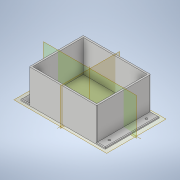
# Autodesk Inventor part: Box
Saved by Autodesk Inventor 2021 (Build 250183000, 183)
## iProperties
Created: 2024-05-07
Part Number: Box
Material: Generisch
Document SubType Name: Modeling
Designer: pasca
Density: 1 g/cm^3
Appearance: Vorgabe
Author: pasca
Autodesk Inventor part; units mm, degrees
sketch "Skizze1" plane through (0, 0, 0) normal (0, 0, 1) x (1, 0, 0)
  line L0 (-100, 80) -> (100, 80)
  line L1 (100, 80) -> (100, -80)
  line L2 (100, -80) -> (-100, -80)
  line L3 (-100, -80) -> (-100, 80)
  line L4 (0, -112) -> (0, 112) projected
  line L5 (-140, 0) -> (140, 0) projected
  point P0 (0, 0)
  dimension "d0" = 160
  dimension "d1" = 200
  constraints: 8 end point, 2 parallel, 1 horizontal, 1 perpendicular, 2 other
  measures "d0" distance between parallel lines of L2 L0
  measures "d1" distance between parallel lines of L1 L3
extrude "Extrusion1" add sketch "Skizze1" along normal blind 100
sketch "Skizze2" plane through (0, 0, 100) normal (0, 0, 1) x (1, 0, 0)
  line L0 (-95, 75) -> (95, 75)
  line L1 (95, 75) -> (95, -75)
  line L2 (95, -75) -> (-95, -75)
  line L3 (-95, -75) -> (-95, 75)
  line L4 (0, -112) -> (0, 112) projected
  line L5 (-140, 0) -> (140, 0) projected
  point P0 (0, 0)
  dimension "d4" = 150
  dimension "d5" = 190
  constraints: 8 end point, 2 parallel, 1 horizontal, 1 perpendicular, 2 other
  measures "d4" distance between parallel lines of L2 L0
  measures "d5" distance between parallel lines of L1 L3
extrude "Extrusion2" cut sketch "Skizze2" against normal blind 95
sketch "Skizze3" plane through (0, 0, 5) normal (0, 0, 1) x (1, 0, 0)
  line L0 (100, -80) -> (100, 80) projected
  line L1 (100, -80) -> (125, -80)
  line L2 (125, -80) -> (125, 80)
  line L3 (125, 80) -> (100, 80)
  line L4 (100, 80) -> (100, -80)
  point P0 (0, 0)
  constraints: 8 end point, 2 parallel, 1 horizontal, 1 perpendicular
extrude "Extrusion3" add sketch "Skizze3" against normal blind 5
sketch "Skizze4" plane through (0, 0, 5) normal (0, 0, 1) x (1, 0, 0)
  point P0 (0, 0)
sketch "Skizze5" plane through (0, 0, 5) normal (0, 0, 1) x (1, 0, 0)
  line L0 (100, -80) -> (100, 80) projected
  line L1 (100, -80) -> (125, -80) projected
  line L2 (125, -80) -> (125, 80) projected
  line L3 (125, 80) -> (100, 80) projected
  point P0 (0, 0)
  point P1 (112.5, 55)
  point P2 (112.5, -55)
hole "Bohrung2" at (112.5, 55, 5) at (112.5, -55, 5) direction (0, 0, -1) diameter 6.4 depth 8 tip angle 118
mirror "Spiegeln1" about plane through (0, 0, 0) normal (1, 0, 0) of "Extrusion3", "Bohrung2"
fillet "Rundung1" radius 2 10 edges at (125, 0, 5) (-125, 0, 5) (-112.5, -80, 5) (-100, -80, 52.5) (112.5, -80, 5) (100, -80, 52.5) (112.5, 80, 5) (-112.5, 80, 5) (-100, 80, 52.5) (100, 80, 52.5)
